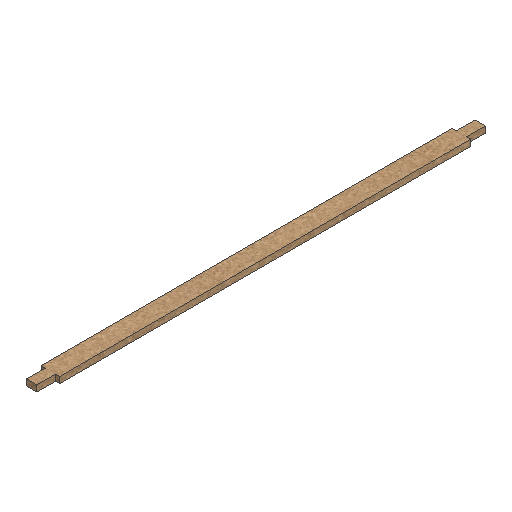
# Autodesk Inventor part: side_Bar
Saved by Autodesk Inventor 2024 (Build 280153000, 153)
## iProperties
Created: 2024-04-09
Part Number: side_Bar
Material: MDF Medium Density Fiberboard
Document SubType Name: Modeling
Designer: USER
Density: 0.8 g/cm^3
Appearance: Cardboard - Corrugated
Mass: 4.5036 g
Surface Area: 51.06 cm^2
Volume: 5.6295 cm^3
Author: USER
Autodesk Inventor part; units mm, degrees
ref_plane "YZ Plane" through (0, 0, 0) normal (1, 0, 0) x (0, 1, 0)
ref_plane "XZ Plane" through (0, 0, 0) normal (0, 1, 0) x (-1, 0, 0)
ref_plane "XY Plane" through (0, 0, 0) normal (0, 0, 1) x (1, 0, 0)
sketch "草圖1" plane through (0, 0, 0) normal (0, 1, 0) x (-1, 0, 0)
  line L0 (0, 0) -> (9, 0)
  line L1 (9, 0) -> (9, -198.5)
  line L2 (9, -198.5) -> (0, -198.5)
  line L3 (0, -198.5) -> (0, 0)
  line L4 (7, 0) -> (2, 0)
  line L5 (2, 0) -> (2, 9)
  line L6 (2, 9) -> (7, 9)
  line L7 (7, 9) -> (7, 0)
  line L8 (7, -198.5) -> (2, -198.5)
  line L9 (2, -198.5) -> (2, -207.5)
  line L10 (2, -207.5) -> (7, -207.5)
  line L11 (7, -207.5) -> (7, -198.5)
  point P0 (4.5, 0)
  point P1 (4.5, -198.5)
  dimension "d0" = 198.5
  dimension "d1" = 9
  dimension "d2" = 9
  dimension "d3" = 5
  dimension "d4" = 9
  dimension "d5" = 5
  constraints: 24 end point, 6 parallel, 4 midpoint, 3 horizontal, 3 perpendicular
  measures "d0" distance of L0.end L1.end
  measures "d1" distance of L0.start L0.end
  measures "d2" distance of L6.end L4.start
  measures "d3" distance of L5.end L6.end
  measures "d4" distance of L10.end L8.start
  measures "d5" distance of L9.end L10.end
extrude "擠出1" add sketch "草圖1" along normal blind 3
